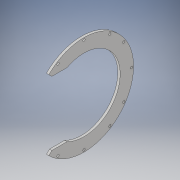
# Autodesk Inventor part: BearingGuard2
Saved by Autodesk Inventor 2018 (Build 220112000, 112)
## iProperties
Created: 2019-02-07
Part Number: BearingGuard2
Material: Generic
Document SubType Name: Modeling
Designer: anirudh
Density: 1 g/cm^3
Appearance: Default
Author: anirudh
Autodesk Inventor part; units mm, degrees
ref_plane "YZ Plane" through (0, 0, 0) normal (1, 0, 0) x (0, 1, 0)
ref_plane "XZ Plane" through (0, 0, 0) normal (0, 1, 0) x (-1, 0, 0)
ref_plane "XY Plane" through (0, 0, 0) normal (0, 0, 1) x (1, 0, 0)
sketch "Sketch5" plane through (0, 0, 0) normal (1, 0, 0) x (0, 1, 0)
  line L0 (-162.5323, -0.9432) -> (-162.5323, -0.9432)
  arc A0 (-167.2919, -5.7027) -> (-55.9367, -5.7027) centre (-111.6143, 49.9749) ccw
  arc A1 (-167.2919, -5.7027) -> (-55.9367, -5.7027) centre (-111.6143, 49.9749) ccw
  circle A2 centre (-70.4577, -13.1714) radius 1.85
  circle A3 centre (-70.4577, -13.1714) radius 1.85
  circle A4 centre (-111.6143, -25.3996) radius 1.85
  circle A5 centre (-111.6143, -25.3996) radius 1.85
  arc A6 (-154.2443, -12.0527) -> (-151.2974, -12.0527) centre (-152.7709, -13.1714) ccw
  circle A7 centre (-152.7709, -13.1714) radius 1.85
  line L1 (-60.6962, 100.8929) -> (-55.9367, 105.6525)
  arc A8 (-55.9367, -5.7027) -> (-55.9367, 105.6525) centre (-111.6143, 49.9749) ccw
  circle A9 centre (-48.468, 91.1314) radius 1.85
  circle A10 centre (-48.468, 91.1314) radius 1.85
  circle A11 centre (-36.2398, 49.9749) radius 1.85
  arc A12 (-49.5867, 7.3449) -> (-49.5867, 10.2918) centre (-48.468, 8.8183) ccw
  circle A13 centre (-48.468, 8.8183) radius 1.85
  line L2 (-162.5323, 100.8929) -> (-162.5323, 100.8929)
  line L3 (-167.2919, 105.6525) -> (-162.5323, 100.8929)
  line L4 (-162.5323, 100.8929) -> (-167.2919, 105.6525)
  line L5 (-162.5323, 76.7356) -> (-162.5323, 100.8929)
  arc A14 (-167.2919, 105.6525) -> (-167.2919, -5.7027) centre (-111.6143, 49.9749) ccw
  arc A15 (-167.2919, 105.6525) -> (-167.2919, -5.7027) centre (-111.6143, 49.9749) ccw
  circle A16 centre (-174.7606, 8.8183) radius 1.85
  circle A17 centre (-174.7606, 8.8183) radius 1.85
  circle A18 centre (-186.9888, 49.9749) radius 1.85
  circle A19 centre (-186.9888, 49.9749) radius 1.85
  arc A20 (-173.6419, 92.6049) -> (-173.6419, 89.658) centre (-174.7606, 91.1314) ccw
  circle A21 centre (-174.7606, 91.1314) radius 1.85
  arc A22 (-162.5323, 76.7356) -> (-60.6962, 76.7356) centre (-111.6143, 49.9749) ccw
  line L6 (-60.6962, 100.8929) -> (-60.6962, 76.7356)
  line L7 (-55.9367, 105.6525) -> (-60.6962, 100.8929)
  line L8 (-60.6962, 100.8929) -> (-60.6962, 76.7356)
  line L9 (-167.2919, 105.6525) -> (-162.5323, 100.8929)
  line L10 (-162.5323, 100.8929) -> (-162.5323, 76.7356)
  arc A23 (-167.2919, 105.6525) -> (-55.9367, 105.6525) centre (-111.6143, 49.9749) ccw
  arc A24 (-162.5323, 76.7356) -> (-60.6962, 76.7356) centre (-111.6143, 49.9749) ccw
  point P0 (0, 0)
  constraints: 25 centre point, 22 end point, 22 point on circle, 9 coincident, 5 collinear, 2 concentric
extrude "Extrusion5" add sketch "Sketch5" along normal blind 3.81
body "Solid2"
